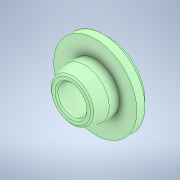
# Autodesk Inventor part: encoder_codewheel_pwb_mount
Saved by Autodesk Inventor 2022.2 (Build 262287000, 287)
## iProperties
Created: 2019-07-04
Part Number: encoder_codewheel_pwb_mount
Material: Generic
Document SubType Name: Modeling
Designer: Jochen
Density: 1 g/cm^3
Appearance: Default
Sending System: SolidWorks 2017
Last Author: Felix
Last Saved: 2021-02-23
Author: Jochen
Autodesk Inventor part; units mm, degrees
ref_plane "YZ Plane" through (0, 0, 0) normal (1, 0, 0) x (0, 1, 0)
ref_plane "XZ Plane" through (0, 0, 0) normal (0, 1, 0) x (-1, 0, 0)
ref_plane "Work Plane3" through (0, 0, 15) normal (0, 0, 1) x (1, 0, 0)
sketch "Sketch1" plane through (0, 0, 15) normal (0, 0, 1) x (1, 0, 0)
  line L0 (-8.4, 0) -> (8.4, 0) construction
  line L1 (0, -8.4) -> (0, 8.4) construction
  circle A0 centre (0, 0) radius 2.1
  circle A1 centre (0, 0) radius 3.5
  circle A2 centre (0, 0) radius 6
  arc A3 (0.3976, 3.7246) -> (0.5788, 3.8401) centre (0.3976, 3.9246) ccw
  line L2 (0.5788, 3.8401) -> (0.7363, 4.1779)
  arc A4 (1.0807, 4.3422) -> (0.7363, 4.1779) centre (1.0082, 4.0511) ccw
  arc A5 (1.2352, 4.3008) -> (1.0807, 4.3422) centre (0, 0) ccw
  arc A6 (1.4512, 3.9863) -> (1.2352, 4.3008) centre (1.1524, 4.0124) ccw
  line L3 (1.4512, 3.9863) -> (1.4188, 3.6151)
  arc A7 (1.4188, 3.6151) -> (1.518, 3.4244) centre (1.618, 3.5976) ccw
  line L4 (1.518, 3.4244) -> (2.2066, 3.0268)
  arc A8 (2.2066, 3.0268) -> (2.4214, 3.0362) centre (2.3066, 3.2001) ccw
  line L5 (2.4214, 3.0362) -> (2.7266, 3.25)
  arc A9 (3.107, 3.2201) -> (2.7266, 3.25) centre (2.8987, 3.0042) ccw
  arc A10 (3.2201, 3.107) -> (3.107, 3.2201) centre (0, 0) ccw
  arc A11 (3.25, 2.7266) -> (3.2201, 3.107) centre (3.0042, 2.8987) ccw
  line L6 (3.25, 2.7266) -> (3.0362, 2.4214)
  arc A12 (3.0362, 2.4214) -> (3.0268, 2.2066) centre (3.2001, 2.3066) ccw
  line L7 (3.0268, 2.2066) -> (3.4244, 1.518)
  arc A13 (3.4244, 1.518) -> (3.6151, 1.4188) centre (3.5976, 1.618) ccw
  line L8 (3.6151, 1.4188) -> (3.9863, 1.4512)
  arc A14 (4.3008, 1.2352) -> (3.9863, 1.4512) centre (4.0124, 1.1524) ccw
  arc A15 (4.3422, 1.0807) -> (4.3008, 1.2352) centre (0, 0) ccw
  arc A16 (4.1779, 0.7363) -> (4.3422, 1.0807) centre (4.0511, 1.0082) ccw
  line L9 (4.1779, 0.7363) -> (3.8401, 0.5788)
  arc A17 (3.8401, 0.5788) -> (3.7246, 0.3976) centre (3.9246, 0.3976) ccw
  line L10 (3.7246, 0.3976) -> (3.7246, -0.3976)
  arc A18 (3.7246, -0.3976) -> (3.8401, -0.5788) centre (3.9246, -0.3976) ccw
  line L11 (3.8401, -0.5788) -> (4.1779, -0.7363)
  arc A19 (4.3422, -1.0807) -> (4.1779, -0.7363) centre (4.0511, -1.0082) ccw
  arc A20 (4.3008, -1.2352) -> (4.3422, -1.0807) centre (0, 0) ccw
  arc A21 (3.9863, -1.4512) -> (4.3008, -1.2352) centre (4.0124, -1.1524) ccw
  line L12 (3.9863, -1.4512) -> (3.6151, -1.4188)
  arc A22 (3.6151, -1.4188) -> (3.4244, -1.518) centre (3.5976, -1.618) ccw
  line L13 (3.4244, -1.518) -> (3.0268, -2.2066)
  arc A23 (3.0268, -2.2066) -> (3.0362, -2.4214) centre (3.2001, -2.3066) ccw
  line L14 (3.0362, -2.4214) -> (3.25, -2.7266)
  arc A24 (3.2201, -3.107) -> (3.25, -2.7266) centre (3.0042, -2.8987) ccw
  arc A25 (3.107, -3.2201) -> (3.2201, -3.107) centre (0, 0) ccw
  arc A26 (2.7266, -3.25) -> (3.107, -3.2201) centre (2.8987, -3.0042) ccw
  line L15 (2.7266, -3.25) -> (2.4214, -3.0362)
  arc A27 (2.4214, -3.0362) -> (2.2066, -3.0268) centre (2.3066, -3.2001) ccw
  line L16 (2.2066, -3.0268) -> (1.518, -3.4244)
  arc A28 (1.518, -3.4244) -> (1.4188, -3.6151) centre (1.618, -3.5976) ccw
  line L17 (1.4188, -3.6151) -> (1.4512, -3.9863)
  arc A29 (1.2352, -4.3008) -> (1.4512, -3.9863) centre (1.1524, -4.0124) ccw
  arc A30 (1.0807, -4.3422) -> (1.2352, -4.3008) centre (0, 0) ccw
  arc A31 (0.7363, -4.1779) -> (1.0807, -4.3422) centre (1.0082, -4.0511) ccw
  line L18 (0.7363, -4.1779) -> (0.5788, -3.8401)
  arc A32 (0.5788, -3.8401) -> (0.3976, -3.7246) centre (0.3976, -3.9246) ccw
  line L19 (0.3976, -3.7246) -> (-0.3976, -3.7246)
  arc A33 (-0.3976, -3.7246) -> (-0.5788, -3.8401) centre (-0.3976, -3.9246) ccw
  line L20 (-0.5788, -3.8401) -> (-0.7363, -4.1779)
  arc A34 (-1.0807, -4.3422) -> (-0.7363, -4.1779) centre (-1.0082, -4.0511) ccw
  arc A35 (-1.2352, -4.3008) -> (-1.0807, -4.3422) centre (0, 0) ccw
  arc A36 (-1.4512, -3.9863) -> (-1.2352, -4.3008) centre (-1.1524, -4.0124) ccw
  line L21 (-1.4512, -3.9863) -> (-1.4188, -3.6151)
  arc A37 (-1.4188, -3.6151) -> (-1.518, -3.4244) centre (-1.618, -3.5976) ccw
  line L22 (-1.518, -3.4244) -> (-2.2066, -3.0268)
  arc A38 (-2.2066, -3.0268) -> (-2.4214, -3.0362) centre (-2.3066, -3.2001) ccw
  line L23 (-2.4214, -3.0362) -> (-2.7266, -3.25)
  arc A39 (-3.107, -3.2201) -> (-2.7266, -3.25) centre (-2.8987, -3.0042) ccw
  arc A40 (-3.2201, -3.107) -> (-3.107, -3.2201) centre (0, 0) ccw
  arc A41 (-3.25, -2.7266) -> (-3.2201, -3.107) centre (-3.0042, -2.8987) ccw
  line L24 (-3.25, -2.7266) -> (-3.0362, -2.4214)
  arc A42 (-3.0362, -2.4214) -> (-3.0268, -2.2066) centre (-3.2001, -2.3066) ccw
  line L25 (-3.0268, -2.2066) -> (-3.4244, -1.518)
  arc A43 (-3.4244, -1.518) -> (-3.6151, -1.4188) centre (-3.5976, -1.618) ccw
  line L26 (-3.6151, -1.4188) -> (-3.9863, -1.4512)
  arc A44 (-4.3008, -1.2352) -> (-3.9863, -1.4512) centre (-4.0124, -1.1524) ccw
  arc A45 (-4.3422, -1.0807) -> (-4.3008, -1.2352) centre (0, 0) ccw
  arc A46 (-4.1779, -0.7363) -> (-4.3422, -1.0807) centre (-4.0511, -1.0082) ccw
  line L27 (-4.1779, -0.7363) -> (-3.8401, -0.5788)
  arc A47 (-3.8401, -0.5788) -> (-3.7246, -0.3976) centre (-3.9246, -0.3976) ccw
  line L28 (-3.7246, -0.3976) -> (-3.7246, 0.3976)
  arc A48 (-3.7246, 0.3976) -> (-3.8401, 0.5788) centre (-3.9246, 0.3976) ccw
  line L29 (-3.8401, 0.5788) -> (-4.1779, 0.7363)
  arc A49 (-4.3422, 1.0807) -> (-4.1779, 0.7363) centre (-4.0511, 1.0082) ccw
  arc A50 (-4.3008, 1.2352) -> (-4.3422, 1.0807) centre (0, 0) ccw
  arc A51 (-3.9863, 1.4512) -> (-4.3008, 1.2352) centre (-4.0124, 1.1524) ccw
  line L30 (-3.9863, 1.4512) -> (-3.6151, 1.4188)
  arc A52 (-3.6151, 1.4188) -> (-3.4244, 1.518) centre (-3.5976, 1.618) ccw
  line L31 (-3.4244, 1.518) -> (-3.0268, 2.2066)
  arc A53 (-3.0268, 2.2066) -> (-3.0362, 2.4214) centre (-3.2001, 2.3066) ccw
  line L32 (-3.0362, 2.4214) -> (-3.25, 2.7266)
  arc A54 (-3.2201, 3.107) -> (-3.25, 2.7266) centre (-3.0042, 2.8987) ccw
  arc A55 (-3.107, 3.2201) -> (-3.2201, 3.107) centre (0, 0) ccw
  arc A56 (-2.7266, 3.25) -> (-3.107, 3.2201) centre (-2.8987, 3.0042) ccw
  line L33 (-2.7266, 3.25) -> (-2.4214, 3.0362)
  arc A57 (-2.4214, 3.0362) -> (-2.2066, 3.0268) centre (-2.3066, 3.2001) ccw
  line L34 (-2.2066, 3.0268) -> (-1.518, 3.4244)
  arc A58 (-1.518, 3.4244) -> (-1.4188, 3.6151) centre (-1.618, 3.5976) ccw
  line L35 (-1.4188, 3.6151) -> (-1.4512, 3.9863)
  arc A59 (-1.2352, 4.3008) -> (-1.4512, 3.9863) centre (-1.1524, 4.0124) ccw
  arc A60 (-1.0807, 4.3422) -> (-1.2352, 4.3008) centre (0, 0) ccw
  arc A61 (-0.7363, 4.1779) -> (-1.0807, 4.3422) centre (-1.0082, 4.0511) ccw
  line L36 (-0.7363, 4.1779) -> (-0.5788, 3.8401)
  arc A62 (-0.5788, 3.8401) -> (-0.3976, 3.7246) centre (-0.3976, 3.9246) ccw
  line L37 (-0.3976, 3.7246) -> (0.3976, 3.7246)
  dimension "d3" = 4.2
  dimension "d4" = 7
  dimension "d5" = 12
  constraints: 120 point on circle, 72 end point, 63 centre point, 3 coincident
  measures "d3" diameter of A0
  measures "d4" diameter of A1
  measures "d5" diameter of A2
extrude "Extrusion1" add sketch "Sketch1" against normal blind 3.5 contours A1
extrude "Extrusion2" add sketch "Sketch1" against normal blind 1.16 from surface at -3.5 contours A1 | A2 | A3 L2 A4 A5 A6 L3 A7 L4 A8 L5 A9 A10 A11 L6 A12 L7 A13 L8 A14 A15 A16 L9 A17 L10 A18 L11 A19 A20 A21 L12 A22 L13 A23 L14 A24 A25 A26 L15 A27 L16 A28 L17 A29 A30 A31 L18 A32 L19 A33 L20 A34 A35 A36 L21 A37 L22 A38 L23 A39 A40 A41 L24 A42 L25 A43 L26 A44 A45 A46 L27 A47 L28 A48 L29 A49 A50 A51 L30 A52 L31 A53 L32 A54 A55 A56 L33 A57 L34 A58 L35 A59 A60 A61 L36 A62 L37
extrude "Extrusion4" add sketch "Sketch1" against normal blind 0.8 from surface at -4.66 separate body contours A2
chamfer "Chamfer1" distance 0.8 angle 45 1 edges at (-6, 0, 9.54)
fillet "Fillet1" radius 0.2 1 edges at (-5.2001, 0, 9.54)
chamfer "Chamfer2" distance 0.2 distance2 0.8 1 edges at (-2.1, 0, 10.34) measured on face at (-2.6, 0, 10.34)
chamfer "Chamfer3" distance 0.5 distance2 2 1 edges at (-3.5, 0, 15) measured on face at (-3, 0, 15)
chamfer "Chamfer4" distance 0.2 angle 45 3 edges at (-3, 0, 15) (-2.1, 0, 15) (-2.3, 0, 10.34)
body "Solid1"
body "Solid2"
body "Solid3"
